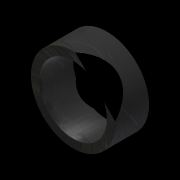
# Autodesk Inventor part: Tread
Saved by Autodesk Inventor 2014 SP1 (Build 180222100, 222)
## iProperties
Created: 2014-05-04
Part Number: Tread
Material: Rubber
Document SubType Name: Modeling
Designer: Rauhul Varma
Mass: 30.2977 g
Surface Area: 125.41 cm^2
Volume: 32.5781 cm^3
Density: 0.93 g/cm^3
Appearance: Rubber - Black - Version 1.1
Author: Rauhul Varma
Autodesk Inventor part; units mm, degrees
ref_plane "YZ Plane" through (0, 0, 0) normal (1, 0, 0) x (0, 1, 0)
ref_plane "XZ Plane" through (0, 0, 0) normal (0, 1, 0) x (-1, 0, 0)
ref_plane "XY Plane" through (0, 0, 0) normal (0, 0, 1) x (1, 0, 0)
sketch "Sketch1" plane through (0, 0, 0) normal (0, 0, 1) x (1, 0, 0)
  circle A0 centre (0, 0) radius 25.4
  circle A1 centre (0, 0) radius 31.75
  dimension "d0" = 50.8
  dimension "d1" = 63.5
  constraints: 2 centre point, 2 coincident
  measures "d0" diameter of A0
  measures "d1" diameter of A1
extrude "Extrusion1" add sketch "Sketch1" along normal mid plane 25.4
body "Solid1"
